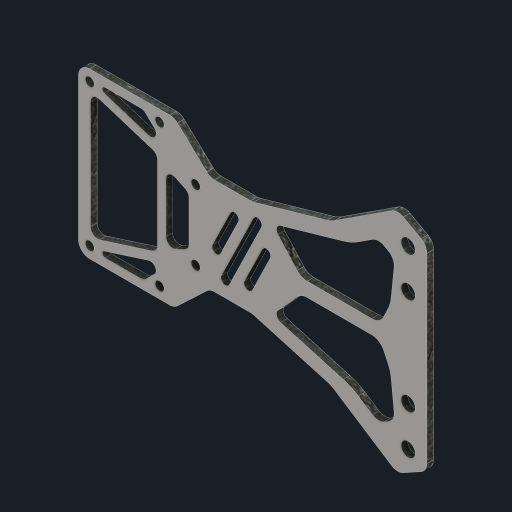
# Autodesk Inventor part: ShoulderBracket2
Saved by Autodesk Inventor 2023 (Build 270158000, 158)
## iProperties
Created: 2021-01-31
Part Number: ShoulderBracket2
Material: Steel
Document SubType Name: Sheet Metal
Designer: valer
Density: 7.85 g/cm^3
Sheet Metal Rule: Default_mm
Appearance: Plate
Mass: 131.888 g
Surface Area: 153.81 cm^2
Volume: 16.801 cm^3
Author: valer
Autodesk Inventor part; units mm, degrees
ref_plane "YZ Plane" through (0, 0, 0) normal (1, 0, 0) x (0, 1, 0)
ref_plane "XZ Plane" through (0, 0, 0) normal (0, 1, 0) x (-1, 0, 0)
ref_plane "XY Plane" through (0, 0, 0) normal (0, 0, 1) x (1, 0, 0)
sketch "Sketch1" plane through (0, 0, 0) normal (0, 0, 1) x (1, 0, 0)
  line L0 (-30.7756, 27.6953) -> (-17.6019, 15.2342)
  arc A0 (-30.7756, 27.6953) -> (-34.2665, 29.0848) centre (-34.2665, 24.0048) ccw
  line L1 (-70.3445, 29.0848) -> (-34.2665, 29.0848)
  arc A1 (-70.3445, 29.0848) -> (-75.4245, 24.0048) centre (-70.3445, 24.0048) ccw
  line L2 (-75.4245, -0.0806) -> (-75.4245, 24.0048)
  line L3 (-43.7214, 16.3936) -> (-63.813, 22.7947)
  arc A2 (-63.4274, 25.2748) -> (-63.813, 22.7947) centre (-63.4274, 24.0048) ccw
  line L4 (-63.4274, 25.2748) -> (-47.0956, 25.2748)
  arc A3 (-45.3502, 24.5801) -> (-47.0956, 25.2748) centre (-47.0956, 22.7348) ccw
  line L5 (-45.3502, 24.5801) -> (-41.2049, 20.659)
  arc A4 (-43.7214, 16.3936) -> (-41.2049, 20.659) centre (-42.9503, 18.8138) ccw
  arc A5 (-65.8672, 19.4505) -> (-70.006, 16.4253) centre (-66.831, 16.4253) ccw
  line L6 (-65.8672, 19.4505) -> (-41.9865, 11.8422)
  line L7 (-70.006, -0.0806) -> (-70.006, 16.4253)
  line L8 (-39.7753, 8.817) -> (-39.7753, -0.0806)
  arc A6 (-39.7753, 8.817) -> (-41.9865, 11.8422) centre (-42.9503, 8.817) ccw
  arc A7 (-17.6019, 15.2342) -> (-14.111, 13.8448) centre (-14.111, 18.9248) ccw
  line L9 (-14.111, 13.8448) -> (2.2031, 13.8448)
  line L10 (3.6033, 14.0416) -> (36.6802, 23.5262)
  arc A8 (2.2031, 13.8448) -> (3.6033, 14.0416) centre (2.2031, 18.9248) ccw
  line L11 (40.0965, 25.0831) -> (65.7679, 41.7543)
  arc A9 (36.6802, 23.5262) -> (40.0965, 25.0831) centre (33.1796, 35.7342) ccw
  arc A10 (70.9975, 41.9369) -> (65.7679, 41.7543) centre (68.5347, 37.4939) ccw
  line L12 (70.9975, 41.9369) -> (79.0399, 37.479)
  arc A11 (81.6571, 33.0359) -> (79.0399, 37.479) centre (76.5771, 33.0359) ccw
  line L13 (81.6571, 33.0359) -> (81.6571, -0.0806)
  line L14 (15.7144, 10.9085) -> (43.9523, 19.0056)
  line L15 (50.785, 22.1194) -> (57.1081, 26.2257)
  arc A12 (43.9523, 19.0056) -> (50.785, 22.1194) centre (36.9512, 43.4216) ccw
  arc A13 (15.7144, 10.9085) -> (14.527, 6.7673) centre (16.4146, 8.4669) ccw
  line L16 (24.9604, -4.8202) -> (14.527, 6.7673)
  line L17 (66.8628, 20.3613) -> (65.2538, 5.1137)
  arc A14 (66.8628, 20.3613) -> (64.2734, 25.3353) centre (61.8106, 20.8923) ccw
  line L18 (62.3377, 26.4083) -> (64.2734, 25.3353)
  arc A15 (62.3377, 26.4083) -> (57.1081, 26.2257) centre (59.8749, 21.9652) ccw
  circle A16 centre (73.1904, 31.6694) radius 3.175
  circle A17 centre (73.1904, 13.8894) radius 3.175
  circle A18 centre (-38.8445, 24.0048) radius 2
  circle A19 centre (-70.3445, 24.0048) radius 2
  line L19 (-75.4245, -0.0806) -> (81.6571, -0.0806) construction
  line L20 (-42.9503, 18.8138) -> (-42.9503, 8.817) construction
  line L21 (-90, -7.9952) -> (-25.0945, -7.9952) construction
  circle A20 centre (-70.3445, -39.9952) radius 2
  arc A21 (-75.4245, -39.9952) -> (-70.3445, -45.0752) centre (-70.3445, -39.9952) ccw
  line L22 (-75.4245, -15.9098) -> (-75.4245, -39.9952)
  line L23 (-70.3445, -45.0752) -> (-34.2665, -45.0752)
  circle A22 centre (-38.8445, -39.9952) radius 2
  arc A23 (-34.2665, -45.0752) -> (-30.7756, -43.6858) centre (-34.2665, -39.9952) ccw
  line L24 (-30.7756, -43.6858) -> (-17.6019, -31.2247)
  arc A24 (-14.111, -29.8352) -> (-17.6019, -31.2247) centre (-14.111, -34.9152) ccw
  line L25 (-14.111, -29.8352) -> (2.2031, -29.8352)
  line L26 (-75.4245, -0.0806) -> (-75.4245, -15.9098)
  arc A25 (-63.813, -38.7851) -> (-63.4274, -41.2652) centre (-63.4274, -39.9952) ccw
  arc A26 (-70.006, -32.4157) -> (-65.8672, -35.4409) centre (-66.831, -32.4157) ccw
  line L27 (-70.006, -0.0806) -> (-70.006, -32.4157)
  line L28 (-63.4274, -41.2652) -> (-47.0956, -41.2652)
  line L29 (-65.8672, -35.4409) -> (-41.9865, -27.8326)
  line L30 (-43.7214, -32.384) -> (-63.813, -38.7851)
  arc A27 (-47.0956, -41.2652) -> (-45.3502, -40.5705) centre (-47.0956, -38.7252) ccw
  line L31 (-45.3502, -40.5705) -> (-41.2049, -36.6495)
  arc A28 (-41.9865, -27.8326) -> (-39.7753, -24.8075) centre (-42.9503, -24.8075) ccw
  arc A29 (-41.2049, -36.6495) -> (-43.7214, -32.384) centre (-42.9503, -34.8042) ccw
  line L32 (-39.7753, -24.8075) -> (-39.7753, -0.0806)
  arc A30 (3.6033, -30.032) -> (2.2031, -29.8352) centre (2.2031, -34.9152) ccw
  line L33 (3.6033, -30.032) -> (36.6802, -39.5166)
  arc A31 (79.0399, -53.4694) -> (81.6571, -49.0263) centre (76.5771, -49.0263) ccw
  line L34 (70.9975, -57.9274) -> (79.0399, -53.4694)
  circle A32 centre (73.1904, -47.6598) radius 3.175
  line L35 (40.0965, -41.0736) -> (65.7679, -57.7447)
  arc A33 (65.7679, -57.7447) -> (70.9975, -57.9274) centre (68.5347, -53.4843) ccw
  circle A34 centre (73.1904, -29.8798) radius 3.175
  arc A35 (40.0965, -41.0736) -> (36.6802, -39.5166) centre (33.1796, -51.7247) ccw
  line L36 (81.6571, -49.0263) -> (81.6571, -15.9098)
  line L37 (81.6571, -15.9098) -> (81.6571, -0.0806)
  line L38 (65.2538, 5.1137) -> (60.6034, -4.8202)
  line L39 (60.6034, -4.8202) -> (24.9604, -4.8202)
  line L40 (62.3377, -42.3987) -> (64.2734, -41.3258)
  arc A36 (64.2734, -41.3258) -> (66.8628, -36.3517) centre (61.8106, -36.8827) ccw
  arc A37 (57.1081, -42.2161) -> (62.3377, -42.3987) centre (59.8749, -37.9557) ccw
  line L41 (66.8628, -36.3517) -> (65.2538, -21.1042)
  line L42 (50.785, -38.1098) -> (57.1081, -42.2161)
  arc A38 (50.785, -38.1098) -> (43.9523, -34.996) centre (36.9512, -59.412) ccw
  arc A39 (14.527, -22.7577) -> (15.7144, -26.8989) centre (16.4146, -24.4573) ccw
  line L43 (24.9604, -11.1702) -> (14.527, -22.7577)
  line L44 (15.7144, -26.8989) -> (43.9523, -34.996)
  line L45 (65.2538, -21.1042) -> (60.6034, -11.1702)
  line L46 (60.6034, -11.1702) -> (24.9604, -11.1702)
  circle A40 centre (-38.8445, -39.9952) radius 2 construction
  circle A41 centre (-22.5945, 7.7548) radius 2
  circle A42 centre (-22.5945, -23.7452) radius 2
  point P0 (0, 0)
  dimension "d0" = 3.175
  dimension "d1" = 3.175
  dimension "d2" = 2.54
  dimension "d3" = 1.27
  dimension "d4" = 2.54
  dimension "d5" = 4
  dimension "d6" = 72.328
  dimension "d11" = 3.81
  dimension "d12" = 16.3318
  dimension "d13" = 3.4035
  dimension "d14" = 7.5795
  dimension "d16" = 3.81
  dimension "d18" = 5.4186
  dimension "d29" = 6.35
  dimension "d30" = 6.35
  dimension "d31" = 16.4032
  dimension "d32" = 21.0537
  measures "d0" radius of A5
  measures "d1" radius of A6
  measures "d2" radius of A4
  measures "d3" radius of A2
  measures "d4" radius of A3
  measures "d5" diameter of A19
  measures "d6" angle of L7 L6
  measures "d11" distance between parallel lines of L1 L4
  measures "d12" distance of L4.start L4.end
  measures "d13" horizontal distance of A5.centre A2.centre
  measures "d14" vertical distance of A2.centre A5.centre
  measures "d16" distance between parallel lines of L6 L3
  measures "d18" distance between parallel lines of L2 L7
  measures "d29" distance between parallel lines of L10 L14
  measures "d30" distance between parallel lines of L46 L39
  measures "d31" distance from line of L13 L17.end
  measures "d32" distance from line of L37 L38.end
extrude "Plate1" add sketch "Sketch1" along normal blind 3
sketch "Sketch2" plane through (0, 0, 3) normal (0, 0, 1) x (1, 0, 0)
  line L0 (-35.9653, 8.0048) -> (-25.5945, 3.0983)
  line L1 (-25.5945, 3.0983) -> (-25.5945, -19.0888)
  line L2 (-25.5945, -19.0888) -> (-35.9653, -23.9952)
  line L3 (-35.9653, -23.9952) -> (-35.9653, 8.0048)
  line L4 (-39.7753, 8.817) -> (-39.7753, -24.8075) construction
  line L5 (-39.7753, -24.8075) -> (-39.7753, 8.817) construction
  line L6 (-39.7753, -7.9952) -> (-35.9653, -7.9952) construction
  line L7 (-65.8672, 19.4505) -> (-41.9865, 11.8422) projected
  line L8 (-43.7214, 16.3936) -> (-63.813, 22.7947) projected
  circle A0 centre (-22.5945, 7.7548) radius 2 construction
  circle A1 centre (-22.5945, -23.7452) radius 2 construction
  line L9 (-22.5945, 7.7548) -> (-22.5945, -23.7452) construction
  circle A2 centre (-22.5945, 7.7548) radius 5.25 construction
  point P0 (0, 0)
  dimension "d20" = 3.81
  dimension "d21" = 3.81
  dimension "d22" = 64.681
  dimension "d23" = 64.681
  dimension "d44" = 32
  dimension "d45" = 3
  dimension "d46" = 10.5
  constraints: 12 end point, 2 midpoint, 2 vertical, 1 centre point, 1 coincident, 1 equal length, 1 parallel, 1 perpendicular
  measures "d20" distance between parallel lines of L7 L8
  measures "d21" distance between parallel lines of L4 L3
  measures "d22" angle of L0 L3
  measures "d23" angle of L3 L2
  measures "d44" distance of L2.end L0.start
  measures "d45" distance between parallel lines of L9 L1
  measures "d46" diameter of A2
extrude "Extrusion1" cut sketch "Sketch2" against normal blind 10
fillet "Fillet1" radius 3 4 edges at (-35.9653, 8.0048, 1.5) (-25.5945, 3.0983, 1.5) (-25.5945, -19.0888, 1.5) (-35.9653, -23.9952, 1.5)
fillet "Fillet2" radius 16 2 edges at (65.2538, 5.1137, 1.5) (65.2538, -21.1042, 1.5)
fillet "Fillet3" radius 6 4 edges at (60.6034, -4.8202, 1.5) (24.9604, -4.8202, 1.5) (24.9604, -11.1702, 1.5) (60.6034, -11.1702, 1.5)
sketch "Sketch4" plane through (0, 0, 3) normal (0, 0, 1) x (1, 0, 0)
  line L0 (-13.1785, -12.7253) -> (-5.1435, 3.7488) construction
  line L1 (-11.3809, -13.602) -> (-3.3459, 2.8721)
  line L2 (-6.9411, 4.6255) -> (-14.9761, -11.8486)
  arc A0 (-14.9761, -11.8486) -> (-11.3809, -13.602) centre (-13.1785, -12.7253) ccw
  arc A1 (-3.3459, 2.8721) -> (-6.9411, 4.6255) centre (-5.1435, 3.7488) ccw
  line L3 (-9.2038, -22.8253) -> (5.2625, 6.8349) construction
  line L4 (-11.0013, -21.9486) -> (3.4649, 7.7116)
  line L5 (7.0601, 5.9581) -> (-7.4062, -23.7021)
  arc A2 (-11.0013, -21.9486) -> (-7.4062, -23.7021) centre (-9.2038, -22.8253) ccw
  arc A3 (7.0601, 5.9581) -> (3.4649, 7.7116) centre (5.2625, 6.8349) ccw
  line L6 (1.2022, -19.7392) -> (9.2372, -3.2651) construction
  line L7 (-0.5953, -18.8625) -> (7.4396, -2.3884)
  line L8 (11.0348, -4.1419) -> (2.9998, -20.616)
  arc A4 (-0.5953, -18.8625) -> (2.9998, -20.616) centre (1.2022, -19.7392) ccw
  arc A5 (11.0348, -4.1419) -> (7.4396, -2.3884) centre (9.2372, -3.2651) ccw
  line L9 (-25.5945, 1.1988) -> (-25.5945, -17.1893) projected
  line L10 (-9.161, -4.4882) -> (5.2197, -11.5022) construction
  line L11 (-14.111, 13.8448) -> (2.2031, 13.8448) construction
  line L12 (2.2031, -29.8352) -> (-14.111, -29.8352) construction
  point P0 (0, 0)
  point P1 (-1.9706, -7.9952)
  point P2 (-1.9706, -7.9952)
  dimension "d37" = 26
  dimension "d38" = 7.0099
  dimension "d39" = 7.0099
  dimension "d40" = 4
  dimension "d41" = 4
  dimension "d47" = 33
  constraints: 26 end point, 12 point on circle, 12 tangent, 6 centre point, 6 midpoint, 6 parallel, 2 equal radius, 1 perpendicular, 1 other
  measures "d37" angle of L9 L0
  measures "d38" distance from line of L11 L3.end
  measures "d39" distance from line of L12 L3.start
  measures "d40" distance between parallel lines of L4 L1
  measures "d41" distance between parallel lines of L7 L5
  measures "d47" distance of L3.start L3.end
extrude "Extrusion3" cut sketch "Sketch4" against normal blind 10
equation "\"d21\" = d20"
equation "\"d23\" = d22"
equation "\"d19\" = Thickness"
equation "\"BendRadius\" = Thickness"
equation "\"BendReliefWidth\" = Thickness"
equation "\"BendReliefDepth\" = 0.5 * Thickness"
equation "\"CornerReliefSize\" = 4 * Thickness"
equation "\"MinimumRemnant\" = 2 * Thickness"
equation "\"TransitionRadius\" = BendRadius"
equation "\"JacobiRadiusSize\" = BendRadius"
equation "\"GapSize\" = Thickness"
equation "\"Thickness\" = 3"
body "Solid1"
